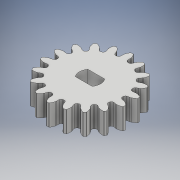
# Autodesk Inventor part: RescueKit-Gear-18
Saved by Autodesk Inventor 2018.3 (Build 223284000, 284)
## iProperties
Created: 2019-03-13
Part Number: RescueKit-Gear-18
Material: 一般
Document SubType Name: Modeling
Designer: shun2
Density: 1 g/cm^3
Appearance: 既定
Author: shun2
Autodesk Inventor part; units mm, degrees
ref_plane "YZ Plane" through (0, 0, 0) normal (1, 0, 0) x (0, 1, 0)
ref_plane "XZ Plane" through (0, 0, 0) normal (0, 1, 0) x (-1, 0, 0)
ref_plane "XY Plane" through (0, 0, 0) normal (0, 0, 1) x (1, 0, 0)
sketch "スケッチ1" plane through (0, 0, 0) normal (0, 0, 1) x (1, 0, 0)
  arc A0 (9.805, -1.9651) -> (9.8858, -1.507) centre (0, 0) ccw
  arc A1 (9.8858, -1.507) -> (9.859, -1.4225) centre (9.7869, -1.4919) ccw
  arc A2 (9.859, -1.4225) -> (8.9658, -0.7844) centre (7.6979, -3.5033) ccw
  arc A3 (8.9658, -0.7844) -> (8.707, -0.7127) centre (8.6226, -1.5204) ccw
  arc A4 (8.0844, -0.573) -> (8.707, -0.7127) centre (8.9979, 2.0412) ccw
  arc A5 (7.7494, -0.0949) -> (8.0844, -0.573) centre (8.2494, -0.101) ccw
  arc A6 (7.7494, -0.0949) -> (7.7494, 0.0949) centre (0, 0) ccw
  arc A7 (8.0844, 0.573) -> (7.7494, 0.0949) centre (8.2494, 0.101) ccw
  arc A8 (8.707, 0.7127) -> (8.0844, 0.573) centre (8.9979, -2.0412) ccw
  arc A9 (8.707, 0.7127) -> (8.9658, 0.7844) centre (8.6226, 1.5204) ccw
  arc A10 (8.9658, 0.7844) -> (9.859, 1.4225) centre (7.6979, 3.5033) ccw
  arc A11 (9.859, 1.4225) -> (9.8858, 1.507) centre (9.7869, 1.4919) ccw
  arc A12 (9.8858, 1.507) -> (9.805, 1.9651) centre (0, 0) ccw
  arc A13 (9.805, 1.9651) -> (9.7509, 2.0352) centre (9.707, 1.9454) ccw
  arc A14 (9.7509, 2.0352) -> (8.6933, 2.3294) centre (8.4319, -0.6592) ccw
  arc A15 (8.6933, 2.3294) -> (8.4257, 2.3082) centre (8.6226, 1.5204) ccw
  arc A16 (7.7929, 2.2266) -> (8.4257, 2.3082) centre (7.7572, 4.9956) ccw
  arc A17 (7.3145, 2.5613) -> (7.7929, 2.2266) centre (7.7864, 2.7265) ccw
  arc A18 (7.3145, 2.5613) -> (7.2496, 2.7396) centre (0, 0) ccw
  arc A19 (7.4009, 3.3035) -> (7.2496, 2.7396) centre (7.7173, 2.9164) ccw
  arc A20 (7.9381, 3.6477) -> (7.4009, 3.3035) centre (9.1534, 1.1594) ccw
  arc A21 (7.9381, 3.6477) -> (8.1568, 3.8036) centre (7.5825, 4.3778) ccw
  arc A22 (8.1568, 3.8036) -> (8.7779, 4.7087) centre (6.0354, 5.9249) ccw
  arc A23 (8.7779, 4.7087) -> (8.7742, 4.7972) centre (8.6865, 4.7492) ccw
  arc A24 (8.7742, 4.7972) -> (8.5416, 5.2001) centre (0, 0) ccw
  arc A25 (8.5416, 5.2001) -> (8.4668, 5.2475) centre (8.4562, 5.1481) ccw
  arc A26 (8.4668, 5.2475) -> (7.3724, 5.1622) centre (8.1488, 2.2644) ccw
  arc A27 (7.3724, 5.1622) -> (7.1281, 5.0508) centre (7.5825, 4.3778) ccw
  arc A28 (6.5614, 4.7576) -> (7.1281, 5.0508) centre (5.5808, 7.3474) ccw
  arc A29 (5.9974, 4.9085) -> (6.5614, 4.7576) centre (6.3843, 5.2252) ccw
  arc A30 (5.9974, 4.9085) -> (5.8754, 5.0539) centre (0, 0) ccw
  arc A31 (5.8247, 5.6356) -> (5.8754, 5.0539) centre (6.2545, 5.38) ccw
  arc A32 (6.2118, 6.1427) -> (5.8247, 5.6356) centre (8.2049, 4.2201) ccw
  arc A33 (6.2118, 6.1427) -> (6.364, 6.364) centre (5.628, 6.7072) ccw
  arc A34 (6.364, 6.364) -> (6.638, 7.4269) centre (3.645, 7.6318) ccw
  arc A35 (6.638, 7.4269) -> (6.6043, 7.5089) centre (6.5383, 7.4338) ccw
  arc A36 (6.6043, 7.5089) -> (6.248, 7.8079) centre (0, 0) ccw
  arc A37 (6.248, 7.8079) -> (6.1614, 7.8269) centre (6.1855, 7.7298) ccw
  arc A38 (6.1614, 7.8269) -> (5.1622, 7.3724) centre (6.8829, 4.9149) ccw
  arc A39 (5.1622, 7.3724) -> (4.9707, 7.1841) centre (5.628, 6.7072) ccw
  arc A40 (4.5385, 6.7148) -> (4.9707, 7.1841) centre (2.7312, 8.813) ccw
  arc A41 (3.9569, 6.6637) -> (4.5385, 6.7148) centre (4.2122, 7.0937) ccw
  arc A42 (3.9569, 6.6637) -> (3.7925, 6.7586) centre (0, 0) ccw
  arc A43 (3.546, 7.2879) -> (3.7925, 6.7586) centre (4.0372, 7.1947) ccw
  arc A44 (3.7363, 7.8968) -> (3.546, 7.2879) centre (6.2667, 6.7718) ccw
  arc A45 (3.7363, 7.8968) -> (3.8036, 8.1568) centre (2.9946, 8.2275) ccw
  arc A46 (3.8036, 8.1568) -> (3.6975, 9.2494) centre (0.815, 8.4182) ccw
  arc A47 (3.6975, 9.2494) -> (3.6378, 9.3148) centre (3.6015, 9.2217) ccw
  arc A48 (3.6378, 9.3148) -> (3.2007, 9.4739) centre (0, 0) ccw
  arc A49 (3.2007, 9.4739) -> (3.1129, 9.4622) centre (3.1687, 9.3792) ccw
  arc A50 (3.1129, 9.4622) -> (2.3294, 8.6933) centre (4.7868, 6.9726) ccw
  arc A51 (2.3294, 8.6933) -> (2.2138, 8.4509) centre (2.9946, 8.2275) ccw
  arc A52 (1.9682, 7.8621) -> (2.2138, 8.4509) centre (-0.4477, 9.2157) ccw
  arc A53 (1.4391, 7.6152) -> (1.9682, 7.8621) centre (1.532, 8.1065) ccw
  arc A54 (1.4391, 7.6152) -> (1.2522, 7.6482) centre (0, 0) ccw
  arc A55 (0.8395, 8.0611) -> (1.2522, 7.6482) centre (1.333, 8.1416) ccw
  arc A56 (0.8101, 8.6985) -> (0.8395, 8.0611) centre (3.5727, 8.5068) ccw
  arc A57 (0.8101, 8.6985) -> (0.7844, 8.9658) centre (0, 8.7556) ccw
  arc A58 (0.7844, 8.9658) -> (0.3111, 9.9562) centre (-2.1134, 8.1893) ccw
  arc A59 (0.3111, 9.9562) -> (0.2326, 9.9973) centre (0.2303, 9.8973) ccw
  arc A60 (0.2326, 9.9973) -> (-0.2326, 9.9973) centre (0, 0) ccw
  arc A61 (-0.2326, 9.9973) -> (-0.3111, 9.9562) centre (-0.2303, 9.8973) ccw
  arc A62 (-0.3111, 9.9562) -> (-0.7844, 8.9658) centre (2.1134, 8.1893) ccw
  arc A63 (-0.7844, 8.9658) -> (-0.8101, 8.6985) centre (0, 8.7556) ccw
  arc A64 (-0.8395, 8.0611) -> (-0.8101, 8.6985) centre (-3.5727, 8.5068) ccw
  arc A65 (-1.2522, 7.6482) -> (-0.8395, 8.0611) centre (-1.333, 8.1416) ccw
  arc A66 (-1.2522, 7.6482) -> (-1.4391, 7.6152) centre (0, 0) ccw
  arc A67 (-1.9682, 7.8621) -> (-1.4391, 7.6152) centre (-1.532, 8.1065) ccw
  arc A68 (-2.2138, 8.4509) -> (-1.9682, 7.8621) centre (0.4477, 9.2157) ccw
  arc A69 (-2.2138, 8.4509) -> (-2.3294, 8.6933) centre (-2.9946, 8.2275) ccw
  arc A70 (-2.3294, 8.6933) -> (-3.1129, 9.4622) centre (-4.7868, 6.9726) ccw
  arc A71 (-3.1129, 9.4622) -> (-3.2007, 9.4739) centre (-3.1687, 9.3792) ccw
  arc A72 (-3.2007, 9.4739) -> (-3.6378, 9.3148) centre (0, 0) ccw
  arc A73 (-3.6378, 9.3148) -> (-3.6975, 9.2494) centre (-3.6015, 9.2217) ccw
  arc A74 (-3.6975, 9.2494) -> (-3.8036, 8.1568) centre (-0.815, 8.4182) ccw
  arc A75 (-3.8036, 8.1568) -> (-3.7363, 7.8968) centre (-2.9946, 8.2275) ccw
  arc A76 (-3.546, 7.2879) -> (-3.7363, 7.8968) centre (-6.2667, 6.7718) ccw
  arc A77 (-3.7925, 6.7586) -> (-3.546, 7.2879) centre (-4.0372, 7.1947) ccw
  arc A78 (-3.7925, 6.7586) -> (-3.9569, 6.6637) centre (0, 0) ccw
  arc A79 (-4.5385, 6.7148) -> (-3.9569, 6.6637) centre (-4.2122, 7.0937) ccw
  arc A80 (-4.9707, 7.1841) -> (-4.5385, 6.7148) centre (-2.7312, 8.813) ccw
  arc A81 (-4.9707, 7.1841) -> (-5.1622, 7.3724) centre (-5.628, 6.7072) ccw
  arc A82 (-5.1622, 7.3724) -> (-6.1614, 7.8269) centre (-6.8829, 4.9149) ccw
  arc A83 (-6.1614, 7.8269) -> (-6.248, 7.8079) centre (-6.1855, 7.7298) ccw
  arc A84 (-6.248, 7.8079) -> (-6.6043, 7.5089) centre (0, 0) ccw
  arc A85 (-6.6043, 7.5089) -> (-6.638, 7.4269) centre (-6.5383, 7.4338) ccw
  arc A86 (-6.638, 7.4269) -> (-6.364, 6.364) centre (-3.645, 7.6318) ccw
  arc A87 (-6.364, 6.364) -> (-6.2118, 6.1427) centre (-5.628, 6.7072) ccw
  arc A88 (-5.8247, 5.6356) -> (-6.2118, 6.1427) centre (-8.2049, 4.2201) ccw
  arc A89 (-5.8754, 5.0539) -> (-5.8247, 5.6356) centre (-6.2545, 5.38) ccw
  arc A90 (-5.8754, 5.0539) -> (-5.9974, 4.9085) centre (0, 0) ccw
  arc A91 (-6.5614, 4.7576) -> (-5.9974, 4.9085) centre (-6.3843, 5.2252) ccw
  arc A92 (-7.1281, 5.0508) -> (-6.5614, 4.7576) centre (-5.5808, 7.3474) ccw
  arc A93 (-7.1281, 5.0508) -> (-7.3724, 5.1622) centre (-7.5825, 4.3778) ccw
  arc A94 (-7.3724, 5.1622) -> (-8.4668, 5.2475) centre (-8.1488, 2.2644) ccw
  arc A95 (-8.4668, 5.2475) -> (-8.5416, 5.2001) centre (-8.4562, 5.1481) ccw
  arc A96 (-8.5416, 5.2001) -> (-8.7742, 4.7972) centre (0, 0) ccw
  arc A97 (-8.7742, 4.7972) -> (-8.7779, 4.7087) centre (-8.6865, 4.7492) ccw
  arc A98 (-8.7779, 4.7087) -> (-8.1568, 3.8036) centre (-6.0354, 5.9249) ccw
  arc A99 (-8.1568, 3.8036) -> (-7.9381, 3.6477) centre (-7.5825, 4.3778) ccw
  arc A100 (-7.4009, 3.3035) -> (-7.9381, 3.6477) centre (-9.1534, 1.1594) ccw
  arc A101 (-7.2496, 2.7396) -> (-7.4009, 3.3035) centre (-7.7173, 2.9164) ccw
  arc A102 (-7.2496, 2.7396) -> (-7.3145, 2.5613) centre (0, 0) ccw
  arc A103 (-7.7929, 2.2266) -> (-7.3145, 2.5613) centre (-7.7864, 2.7265) ccw
  arc A104 (-8.4257, 2.3082) -> (-7.7929, 2.2266) centre (-7.7572, 4.9956) ccw
  arc A105 (-8.4257, 2.3082) -> (-8.6933, 2.3294) centre (-8.6226, 1.5204) ccw
  arc A106 (-8.6933, 2.3294) -> (-9.7509, 2.0352) centre (-8.4319, -0.6592) ccw
  arc A107 (-9.7509, 2.0352) -> (-9.805, 1.9651) centre (-9.707, 1.9454) ccw
  arc A108 (-9.805, 1.9651) -> (-9.8858, 1.507) centre (0, 0) ccw
  arc A109 (-9.8858, 1.507) -> (-9.859, 1.4225) centre (-9.7869, 1.4919) ccw
  arc A110 (-9.859, 1.4225) -> (-8.9658, 0.7844) centre (-7.6979, 3.5033) ccw
  arc A111 (-8.9658, 0.7844) -> (-8.707, 0.7127) centre (-8.6226, 1.5204) ccw
  arc A112 (-8.0844, 0.573) -> (-8.707, 0.7127) centre (-8.9979, -2.0412) ccw
  arc A113 (-7.7494, 0.0949) -> (-8.0844, 0.573) centre (-8.2494, 0.101) ccw
  arc A114 (-7.7494, 0.0949) -> (-7.7494, -0.0949) centre (0, 0) ccw
  arc A115 (-8.0844, -0.573) -> (-7.7494, -0.0949) centre (-8.2494, -0.101) ccw
  arc A116 (-8.707, -0.7127) -> (-8.0844, -0.573) centre (-8.9979, 2.0412) ccw
  arc A117 (-8.707, -0.7127) -> (-8.9658, -0.7844) centre (-8.6226, -1.5204) ccw
  arc A118 (-8.9658, -0.7844) -> (-9.859, -1.4225) centre (-7.6979, -3.5033) ccw
  arc A119 (-9.859, -1.4225) -> (-9.8858, -1.507) centre (-9.7869, -1.4919) ccw
  arc A120 (-9.8858, -1.507) -> (-9.805, -1.9651) centre (0, 0) ccw
  arc A121 (-9.805, -1.9651) -> (-9.7509, -2.0352) centre (-9.707, -1.9454) ccw
  arc A122 (-9.7509, -2.0352) -> (-8.6933, -2.3294) centre (-8.4319, 0.6592) ccw
  arc A123 (-8.6933, -2.3294) -> (-8.4257, -2.3082) centre (-8.6226, -1.5204) ccw
  arc A124 (-7.7929, -2.2266) -> (-8.4257, -2.3082) centre (-7.7572, -4.9956) ccw
  arc A125 (-7.3145, -2.5613) -> (-7.7929, -2.2266) centre (-7.7864, -2.7265) ccw
  arc A126 (-7.3145, -2.5613) -> (-7.2496, -2.7396) centre (0, 0) ccw
  arc A127 (-7.4009, -3.3035) -> (-7.2496, -2.7396) centre (-7.7173, -2.9164) ccw
  arc A128 (-7.9381, -3.6477) -> (-7.4009, -3.3035) centre (-9.1534, -1.1594) ccw
  arc A129 (-7.9381, -3.6477) -> (-8.1568, -3.8036) centre (-7.5825, -4.3778) ccw
  arc A130 (-8.1568, -3.8036) -> (-8.7779, -4.7087) centre (-6.0354, -5.9249) ccw
  arc A131 (-8.7779, -4.7087) -> (-8.7742, -4.7972) centre (-8.6865, -4.7492) ccw
  arc A132 (-8.7742, -4.7972) -> (-8.5416, -5.2001) centre (0, 0) ccw
  arc A133 (-8.5416, -5.2001) -> (-8.4668, -5.2475) centre (-8.4562, -5.1481) ccw
  arc A134 (-8.4668, -5.2475) -> (-7.3724, -5.1622) centre (-8.1488, -2.2644) ccw
  arc A135 (-7.3724, -5.1622) -> (-7.1281, -5.0508) centre (-7.5825, -4.3778) ccw
  arc A136 (-6.5614, -4.7576) -> (-7.1281, -5.0508) centre (-5.5808, -7.3474) ccw
  arc A137 (-5.9974, -4.9085) -> (-6.5614, -4.7576) centre (-6.3843, -5.2252) ccw
  arc A138 (-5.9974, -4.9085) -> (-5.8754, -5.0539) centre (0, 0) ccw
  arc A139 (-5.8247, -5.6356) -> (-5.8754, -5.0539) centre (-6.2545, -5.38) ccw
  arc A140 (-6.2118, -6.1427) -> (-5.8247, -5.6356) centre (-8.2049, -4.2201) ccw
  arc A141 (-6.2118, -6.1427) -> (-6.364, -6.364) centre (-5.628, -6.7072) ccw
  arc A142 (-6.364, -6.364) -> (-6.638, -7.4269) centre (-3.645, -7.6318) ccw
  arc A143 (-6.638, -7.4269) -> (-6.6043, -7.5089) centre (-6.5383, -7.4338) ccw
  arc A144 (-6.6043, -7.5089) -> (-6.248, -7.8079) centre (0, 0) ccw
  arc A145 (-6.248, -7.8079) -> (-6.1614, -7.8269) centre (-6.1855, -7.7298) ccw
  arc A146 (-6.1614, -7.8269) -> (-5.1622, -7.3724) centre (-6.8829, -4.9149) ccw
  arc A147 (-5.1622, -7.3724) -> (-4.9707, -7.1841) centre (-5.628, -6.7072) ccw
  arc A148 (-4.5385, -6.7148) -> (-4.9707, -7.1841) centre (-2.7312, -8.813) ccw
  arc A149 (-3.9569, -6.6637) -> (-4.5385, -6.7148) centre (-4.2122, -7.0937) ccw
  arc A150 (-3.9569, -6.6637) -> (-3.7925, -6.7586) centre (0, 0) ccw
  arc A151 (-3.546, -7.2879) -> (-3.7925, -6.7586) centre (-4.0372, -7.1947) ccw
  arc A152 (-3.7363, -7.8968) -> (-3.546, -7.2879) centre (-6.2667, -6.7718) ccw
  arc A153 (-3.7363, -7.8968) -> (-3.8036, -8.1568) centre (-2.9946, -8.2275) ccw
  arc A154 (-3.8036, -8.1568) -> (-3.6975, -9.2494) centre (-0.815, -8.4182) ccw
  arc A155 (-3.6975, -9.2494) -> (-3.6378, -9.3148) centre (-3.6015, -9.2217) ccw
  arc A156 (-3.6378, -9.3148) -> (-3.2007, -9.4739) centre (0, 0) ccw
  arc A157 (-3.2007, -9.4739) -> (-3.1129, -9.4622) centre (-3.1687, -9.3792) ccw
  arc A158 (-3.1129, -9.4622) -> (-2.3294, -8.6933) centre (-4.7868, -6.9726) ccw
  arc A159 (-2.3294, -8.6933) -> (-2.2138, -8.4509) centre (-2.9946, -8.2275) ccw
  arc A160 (-1.9682, -7.8621) -> (-2.2138, -8.4509) centre (0.4477, -9.2157) ccw
  arc A161 (-1.4391, -7.6152) -> (-1.9682, -7.8621) centre (-1.532, -8.1065) ccw
  arc A162 (-1.4391, -7.6152) -> (-1.2522, -7.6482) centre (0, 0) ccw
  arc A163 (-0.8395, -8.0611) -> (-1.2522, -7.6482) centre (-1.333, -8.1416) ccw
  arc A164 (-0.8101, -8.6985) -> (-0.8395, -8.0611) centre (-3.5727, -8.5068) ccw
  arc A165 (-0.8101, -8.6985) -> (-0.7844, -8.9658) centre (0, -8.7556) ccw
  arc A166 (-0.7844, -8.9658) -> (-0.3111, -9.9562) centre (2.1134, -8.1893) ccw
  arc A167 (-0.3111, -9.9562) -> (-0.2326, -9.9973) centre (-0.2303, -9.8973) ccw
  arc A168 (-0.2326, -9.9973) -> (0.2326, -9.9973) centre (0, 0) ccw
  arc A169 (0.2326, -9.9973) -> (0.3111, -9.9562) centre (0.2303, -9.8973) ccw
  arc A170 (0.3111, -9.9562) -> (0.7844, -8.9658) centre (-2.1134, -8.1893) ccw
  arc A171 (0.7844, -8.9658) -> (0.8101, -8.6985) centre (0, -8.7556) ccw
  arc A172 (0.8395, -8.0611) -> (0.8101, -8.6985) centre (3.5727, -8.5068) ccw
  arc A173 (1.2522, -7.6482) -> (0.8395, -8.0611) centre (1.333, -8.1416) ccw
  arc A174 (1.2522, -7.6482) -> (1.4391, -7.6152) centre (0, 0) ccw
  arc A175 (1.9682, -7.8621) -> (1.4391, -7.6152) centre (1.532, -8.1065) ccw
  arc A176 (2.2138, -8.4509) -> (1.9682, -7.8621) centre (-0.4477, -9.2157) ccw
  arc A177 (2.2138, -8.4509) -> (2.3294, -8.6933) centre (2.9946, -8.2275) ccw
  arc A178 (2.3294, -8.6933) -> (3.1129, -9.4622) centre (4.7868, -6.9726) ccw
  arc A179 (3.1129, -9.4622) -> (3.2007, -9.4739) centre (3.1687, -9.3792) ccw
  arc A180 (3.2007, -9.4739) -> (3.6378, -9.3148) centre (0, 0) ccw
  arc A181 (3.6378, -9.3148) -> (3.6975, -9.2494) centre (3.6015, -9.2217) ccw
  arc A182 (3.6975, -9.2494) -> (3.8036, -8.1568) centre (0.815, -8.4182) ccw
  arc A183 (3.8036, -8.1568) -> (3.7363, -7.8968) centre (2.9946, -8.2275) ccw
  arc A184 (3.546, -7.2879) -> (3.7363, -7.8968) centre (6.2667, -6.7718) ccw
  arc A185 (3.7925, -6.7586) -> (3.546, -7.2879) centre (4.0372, -7.1947) ccw
  arc A186 (3.7925, -6.7586) -> (3.9569, -6.6637) centre (0, 0) ccw
  arc A187 (4.5385, -6.7148) -> (3.9569, -6.6637) centre (4.2122, -7.0937) ccw
  arc A188 (4.9707, -7.1841) -> (4.5385, -6.7148) centre (2.7312, -8.813) ccw
  arc A189 (4.9707, -7.1841) -> (5.1622, -7.3724) centre (5.628, -6.7072) ccw
  arc A190 (5.1622, -7.3724) -> (6.1614, -7.8269) centre (6.8829, -4.9149) ccw
  arc A191 (6.1614, -7.8269) -> (6.248, -7.8079) centre (6.1855, -7.7298) ccw
  arc A192 (6.248, -7.8079) -> (6.6043, -7.5089) centre (0, 0) ccw
  arc A193 (6.6043, -7.5089) -> (6.638, -7.4269) centre (6.5383, -7.4338) ccw
  arc A194 (6.638, -7.4269) -> (6.364, -6.364) centre (3.645, -7.6318) ccw
  arc A195 (6.364, -6.364) -> (6.2118, -6.1427) centre (5.628, -6.7072) ccw
  arc A196 (5.8247, -5.6356) -> (6.2118, -6.1427) centre (8.2049, -4.2201) ccw
  arc A197 (5.8754, -5.0539) -> (5.8247, -5.6356) centre (6.2545, -5.38) ccw
  arc A198 (5.8754, -5.0539) -> (5.9974, -4.9085) centre (0, 0) ccw
  arc A199 (6.5614, -4.7576) -> (5.9974, -4.9085) centre (6.3843, -5.2252) ccw
  arc A200 (7.1281, -5.0508) -> (6.5614, -4.7576) centre (5.5808, -7.3474) ccw
  arc A201 (7.1281, -5.0508) -> (7.3724, -5.1622) centre (7.5825, -4.3778) ccw
  arc A202 (7.3724, -5.1622) -> (8.4668, -5.2475) centre (8.1488, -2.2644) ccw
  arc A203 (8.4668, -5.2475) -> (8.5416, -5.2001) centre (8.4562, -5.1481) ccw
  arc A204 (8.5416, -5.2001) -> (8.7742, -4.7972) centre (0, 0) ccw
  arc A205 (8.7742, -4.7972) -> (8.7779, -4.7087) centre (8.6865, -4.7492) ccw
  arc A206 (8.7779, -4.7087) -> (8.1568, -3.8036) centre (6.0354, -5.9249) ccw
  arc A207 (8.1568, -3.8036) -> (7.9381, -3.6477) centre (7.5825, -4.3778) ccw
  arc A208 (7.4009, -3.3035) -> (7.9381, -3.6477) centre (9.1534, -1.1594) ccw
  arc A209 (7.2496, -2.7396) -> (7.4009, -3.3035) centre (7.7173, -2.9164) ccw
  arc A210 (7.2496, -2.7396) -> (7.3145, -2.5613) centre (0, 0) ccw
  arc A211 (7.7929, -2.2266) -> (7.3145, -2.5613) centre (7.7864, -2.7265) ccw
  arc A212 (8.4257, -2.3082) -> (7.7929, -2.2266) centre (7.7572, -4.9956) ccw
  arc A213 (8.4257, -2.3082) -> (8.6933, -2.3294) centre (8.6226, -1.5204) ccw
  arc A214 (8.6933, -2.3294) -> (9.7509, -2.0352) centre (8.4319, 0.6592) ccw
  arc A215 (9.7509, -2.0352) -> (9.805, -1.9651) centre (9.707, -1.9454) ccw
  line L0 (-2, 1.5) -> (2, 1.5)
  line L1 (2, -1.5) -> (-2, -1.5)
  arc A216 (2, -1.5) -> (2, 1.5) centre (0, 0) ccw
  arc A217 (-2, 1.5) -> (-2, -1.5) centre (0, 0) ccw
  constraints: 436 point on circle, 218 centre point, 4 end point, 1 coincident, 1 horizontal, 1 parallel
extrude "押し出し1" add sketch "スケッチ1" along normal blind 5
